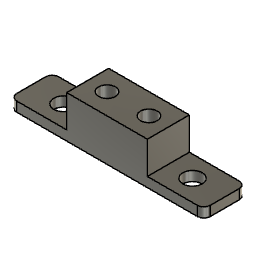
Pos2 (Autodesk Fusion 360 design; units mm, degrees)
Autodesk Fusion 360 part; units mm, degrees
note: some values were not read from the file. Set by a fixed rule: the direction of a hole.
sketch "Sketch1" plane through (0, 0, 0) normal (0, 0, 1) x (1, 0, 0)
  line L0 (28, -6.5) -> (-28, -6.5)
  line L1 (-30, -4.5) -> (-30, 4.5)
  line L2 (-28, 6.5) -> (28, 6.5)
  line L3 (30, 4.5) -> (30, -4.5)
  line L4 (30, -6.5) -> (-30, 6.5) construction
  line L5 (-30, -6.5) -> (30, 6.5) construction
  line L6 (0, 0) -> (20, 0) construction
  line L7 (0, 0) -> (-20, 0) construction
  arc A0 (30, 4.5) -> (28, 6.5) centre (28, 4.5) ccw
  arc A1 (28, -6.5) -> (30, -4.5) centre (28, -4.5) ccw
  arc A2 (-30, -4.5) -> (-28, -6.5) centre (-28, -4.5) ccw
  arc A3 (-28, 6.5) -> (-30, 4.5) centre (-28, 4.5) ccw
  circle A4 centre (20, 0) radius 3
  circle A5 centre (-20, 0) radius 3
  dimension "d1" = 60
  dimension "d2" = 13
  dimension "d3" = 20
  dimension "d4" = 2
  dimension "d5" = 20
  dimension "d6" = 6
  dimension "d7" = 6
  constraint horizontal L0
  constraint perpendicular L0 L1
  constraint parallel L0 L2
  constraint parallel L1 L3
  constraint coincident L4 L6.start
  constraint coincident L5 L6.start
  constraint coincident L6.start L7.start
  constraint parallel L0 L6
  constraint parallel L6 L7
  constraint coincident L5.end L2
  constraint coincident L5.end L3
  constraint tangent L2 A0
  constraint tangent L3 A0
  constraint coincident L4.start L0
  constraint coincident L4.start L3
  constraint tangent L0 A1
  constraint tangent L3 A1
  constraint equal A0 A1
  constraint coincident L5.start L0
  constraint coincident L5.start L1
  constraint tangent L0 A2
  constraint tangent L1 A2
  constraint equal A0 A2
  constraint coincident L4.end L2
  constraint coincident L4.end L1
  constraint tangent L2 A3
  constraint tangent L1 A3
  constraint equal A0 A3
  constraint coincident L6.end A4.centre
  constraint coincident L7.end A5.centre
  measures "d1" distance of L4.end L5.end
  measures "d2" distance of L5.start L4.end
  measures "d3" distance of L6.start L6.end
  measures "d4" radius of A0
  measures "d5" distance of L6.start L7.end
  measures "d6" diameter of A4
  measures "d7" diameter of A5
extrude "Extrude1" add sketch "Sketch1" along normal blind 3
sketch "Sketch2" plane through (0, 0, 3) normal (0, 0, 1) x (-1, 0, 0)
  circle A0 centre (-20, 0) radius 3
  circle A1 centre (20, 0) radius 3
  arc A2 (-30, -4.5) -> (-28, -6.5) centre (-28, -4.5) ccw
  line L0 (-28, -6.5) -> (28, -6.5)
  arc A3 (28, -6.5) -> (30, -4.5) centre (28, -4.5) ccw
  line L1 (30, -4.5) -> (30, 4.5)
  arc A4 (30, 4.5) -> (28, 6.5) centre (28, 4.5) ccw
  line L2 (28, 6.5) -> (-28, 6.5)
  arc A5 (-28, 6.5) -> (-30, 4.5) centre (-28, 4.5) ccw
  line L3 (-30, 4.5) -> (-30, -4.5)
  line L4 (-12.5, 6.5) -> (12.5, 6.5)
  line L5 (12.5, 6.5) -> (12.5, -6.5)
  line L6 (12.5, -6.5) -> (-12.5, -6.5)
  line L7 (-12.5, -6.5) -> (-12.5, 6.5)
  line L8 (-12.5, 6.5) -> (12.5, -6.5) construction
  line L9 (12.5, 6.5) -> (-12.5, -6.5) construction
  line L10 (0, 0) -> (-6.5, 0) construction
  line L11 (0, 0) -> (6.5, 0) construction
  dimension "d10" = 25
  dimension "d11" = 6.5
  dimension "d12" = 6.5
  constraint horizontal L4
  constraint perpendicular L4 L5
  constraint parallel L4 L6
  constraint parallel L5 L7
  constraint coincident L8 L10.start
  constraint coincident L9 L10.start
  constraint coincident L10.start L11.start
  constraint perpendicular L7 L10
  constraint parallel L10 L11
  measures "d10" distance of L5.end L6.end
  measures "d11" distance of L10.start L10.end
  measures "d12" distance of L10.start L11.end
extrude "Extrude2" add sketch "Sketch2" along normal blind 10 contours L0 L2 L4 L5 L6 L7
sketch "Sketch3" plane through (0, 0, 0) normal (0, 0, 1) x (-1, 0, 0)
  line L0 (-12.5, -6.5) -> (12.5, -6.5)
  line L1 (12.5, -6.5) -> (12.5, 6.5)
  line L2 (12.5, 6.5) -> (-12.5, 6.5)
  line L3 (-12.5, 6.5) -> (-12.5, -6.5)
  line L4 (0, 0) -> (-6.5, 0) construction
  line L5 (0, 0) -> (6.5, 0) construction
  circle A0 centre (-6.5, 0) radius 2.6
  line L6 (0, 0) -> (0, -2) construction
  circle A1 centre (6.5, 0) radius 2.6
  circle A2 centre (-20, 0) radius 3
  circle A3 centre (20, 0) radius 3
  arc A4 (-30, -4.5) -> (-28, -6.5) centre (-28, -4.5) ccw
  line L7 (-30, -4.5) -> (-30, 4.5)
  arc A5 (-28, 6.5) -> (-30, 4.5) centre (-28, 4.5) ccw
  line L8 (-28, 6.5) -> (28, 6.5)
  arc A6 (30, 4.5) -> (28, 6.5) centre (28, 4.5) ccw
  line L9 (30, 4.5) -> (30, -4.5)
  arc A7 (28, -6.5) -> (30, -4.5) centre (28, -4.5) ccw
  line L10 (28, -6.5) -> (-28, -6.5)
  dimension "d15" = 6.5
  dimension "d16" = 6.5
  dimension "d17" = 5.2
  dimension "d18" = 2
  constraint coincident L4.start L5.start
  constraint horizontal L4
  constraint parallel L4 L5
  constraint coincident L4.end A0.centre
  constraint perpendicular L4 L6
  constraint symmetric A0 L6 A1
  measures "d15" distance of L4.start L4.end
  measures "d16" distance of L4.start L5.end
  measures "d17" diameter of A0
  measures "d18" distance of L4.start L6.end
hole "Hole1" at (6.5, 0, 0) at (-6.5, 0, 0) direction (0, 0, 1) diameter 5.2 depth 13 tip angle 90 countersink diameter 5.72 countersink angle 90
